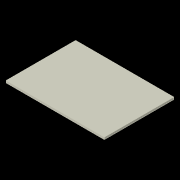
# Autodesk Inventor part: MLMRSMLSMR
Saved by Autodesk Inventor 2016 (Build 200138000, 138)
## iProperties
Created: 2017-01-21
Part Number: MLMRSMLSMR
Material: Generic
Document SubType Name: Modeling
Designer: Alexis Renderos
Density: 1 g/cm^3
Appearance: Ivory Flat
Author: Alexis Renderos
Autodesk Inventor part; units mm, degrees
ref_plane "YZ Plane" through (0, 0, 0) normal (1, 0, 0) x (0, 1, 0)
ref_plane "XZ Plane" through (0, 0, 0) normal (0, 1, 0) x (-1, 0, 0)
ref_plane "XY Plane" through (0, 0, 0) normal (0, 0, 1) x (1, 0, 0)
sketch "Sketch1" plane through (0, 0, 0) normal (0, 1, 0) x (-1, 0, 0)
  line L0 (0, -142.24) -> (0, 142.24) projected
  line L1 (-200.9496, 0) -> (200.9496, 0) projected
  line L2 (143.5354, 101.6) -> (-143.5354, 101.6)
  line L3 (-143.5354, 101.6) -> (-143.5354, -101.6)
  line L4 (-143.5354, -101.6) -> (143.5354, -101.6)
  line L5 (143.5354, -101.6) -> (143.5354, 101.6)
  line L6 (143.5354, 101.6) -> (-143.5354, -101.6) construction
  line L7 (-143.5354, 101.6) -> (143.5354, -101.6) construction
  point P0 (0, 0)
  dimension "d0" = 287.0708
  dimension "d1" = 203.2
  constraints: 12 end point, 2 midpoint, 2 parallel, 1 horizontal, 1 perpendicular
  measures "d0" distance of L4.end L3.end
  measures "d1" distance of L3.end L2.end
extrude "Extrusion1" add sketch "Sketch1" along normal mid plane 6.35
body "Solid1"
